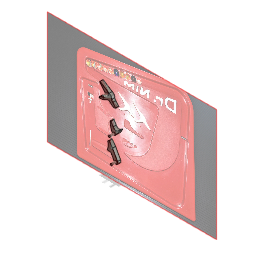
Controls (Autodesk Fusion 360 design; units mm, degrees)
Autodesk Fusion 360 part; units mm, degrees
sketch "Sketch1" plane through (0, 0, 0) normal (0, 0, 1) x (1, 0, 0)
  line L0 (-51.0325, 45.1577) -> (-34.9506, 34.906)
  line L1 (-51.6438, 44.279) -> (-42.8604, 33.3957)
  spline S0 degree 5 poles (-52.4084, 20.9295) (-52.2174, 21.0253) (-51.8369, 21.2159) (-51.271, 21.499) (-50.5262, 21.8709) (-49.6123, 22.3257) (-48.7173, 22.7695) (-47.8428, 23.2013) (-46.9901, 23.6204) (-46.1587, 24.0272) (-45.3471, 24.4223) (-44.7125, 24.7299) (-44.2442, 24.9561) (-43.9354, 25.1049) (-43.7819, 25.1788) knots 0 0 0 0 0 0 0.1 0.2 0.3 0.4 0.5 0.6 0.7 0.8 0.9 1 1 1 1 1 1
  line L2 (-43.6283, 20.7248) -> (-38.8415, 23.1566)
  line L3 (-38.8415, 23.1566) -> (-43.6283, 20.7248)
  line L4 (-28.4743, 24.2061) -> (-23.3292, 18.2162)
  spline S1 degree 5 poles (-42.8604, 33.3957) (-42.7748, 33.2875) (-42.6091, 33.0705) (-42.377, 32.7437) (-42.1008, 32.3051) (-41.8149, 31.7517) (-41.5939, 31.1927) (-41.4431, 30.6277) (-41.3661, 30.0564) (-41.3603, 29.4789) (-41.4207, 28.8958) (-41.5177, 28.4251) (-41.616, 28.0699) (-41.6928, 27.8321) (-41.7341, 27.713) knots 0 0 0 0 0 0 0.1 0.2 0.3 0.4 0.5 0.6 0.7 0.8 0.9 1 1 1 1 1 1
  spline S2 degree 5 poles (-41.7341, 27.713) (-41.759, 27.6465) (-41.8102, 27.515) (-41.8911, 27.3218) (-42.0077, 27.0726) (-42.1685, 26.776) (-42.3458, 26.4956) (-42.5411, 26.2329) (-42.7551, 25.9885) (-42.9871, 25.7619) (-43.2359, 25.5516) (-43.4471, 25.3955) (-43.612, 25.2847) (-43.7248, 25.2136) (-43.7819, 25.1788) knots 0 0 0 0 0 0 0.1 0.2 0.3 0.4 0.5 0.6 0.7 0.8 0.9 1 1 1 1 1 1
  spline S3 degree 5 poles (-43.6283, 20.7248) (-43.7891, 20.6427) (-44.1116, 20.4839) (-44.5982, 20.2616) (-45.2528, 19.9976) (-46.0811, 19.725) (-46.9205, 19.5152) (-47.7719, 19.3729) (-48.6357, 19.301) (-49.5115, 19.2964) (-50.3982, 19.354) (-51.1157, 19.4457) (-51.658, 19.5385) (-52.0214, 19.6108) (-52.2036, 19.6497) knots 0 0 0 0 0 0 0.1 0.2 0.3 0.4 0.5 0.6 0.7 0.8 0.9 1 1 1 1 1 1
  spline S4 degree 5 poles (-52.4084, 20.9295) (-52.4626, 20.896) (-52.5658, 20.8297) (-52.7055, 20.7322) (-52.8605, 20.6065) (-52.9991, 20.4569) (-53.0773, 20.3155) (-53.0905, 20.1829) (-53.0359, 20.0596) (-52.9164, 19.9451) (-52.7369, 19.8387) (-52.5492, 19.7596) (-52.3853, 19.7034) (-52.2658, 19.6673) (-52.2036, 19.6497) knots 0 0 0 0 0 0 0.1 0.2 0.3 0.4 0.5 0.6 0.7 0.8 0.9 1 1 1 1 1 1
  spline S5 degree 5 poles (-38.8415, 23.1566) (-38.7144, 23.2222) (-38.461, 23.3447) (-38.083, 23.5021) (-37.5831, 23.6584) (-36.9658, 23.7583) (-36.3565, 23.7549) (-35.756, 23.6407) (-35.1644, 23.4129) (-34.5812, 23.0779) (-34.0058, 22.6444) (-33.551, 22.2256) (-33.213, 21.8736) (-32.9889, 21.6224) (-32.8772, 21.4927) knots 0 0 0 0 0 0 0.1 0.2 0.3 0.4 0.5 0.6 0.7 0.8 0.9 1 1 1 1 1 1
  spline S6 degree 5 poles (-32.8772, 21.4927) (-32.7115, 21.3178) (-32.3789, 20.9756) (-31.8763, 20.4844) (-31.1986, 19.8749) (-30.3379, 19.1937) (-29.4624, 18.6011) (-28.5707, 18.105) (-27.6619, 17.7112) (-26.7363, 17.4175) (-25.795, 17.2172) (-25.0304, 17.126) (-24.4509, 17.094) (-24.0619, 17.0886) (-23.8667, 17.0899) knots 0 0 0 0 0 0 0.1 0.2 0.3 0.4 0.5 0.6 0.7 0.8 0.9 1 1 1 1 1 1
  spline S7 degree 5 poles (-23.3292, 18.2162) (-23.2856, 18.1711) (-23.2033, 18.083) (-23.094, 17.9567) (-22.9773, 17.8003) (-22.8831, 17.6263) (-22.8451, 17.4756) (-22.8678, 17.3501) (-22.9535, 17.2507) (-23.0996, 17.1764) (-23.3014, 17.1252) (-23.5037, 17.1012) (-23.677, 17.0921) (-23.8019, 17.09) (-23.8667, 17.0899) knots 0 0 0 0 0 0 0.1 0.2 0.3 0.4 0.5 0.6 0.7 0.8 0.9 1 1 1 1 1 1
  spline S8 degree 5 poles (-51.6438, 44.279) (-51.6575, 44.3127) (-51.6828, 44.3788) (-51.7139, 44.4736) (-51.7415, 44.5913) (-51.7512, 44.7232) (-51.7341, 44.8384) (-51.6879, 44.9355) (-51.6115, 45.0139) (-51.5061, 45.0744) (-51.3741, 45.1182) (-51.2489, 45.1411) (-51.1446, 45.1519) (-51.0706, 45.1562) (-51.0325, 45.1577) knots 0 0 0 0 0 0 0.1 0.2 0.3 0.4 0.5 0.6 0.7 0.8 0.9 1 1 1 1 1 1
  spline S9 degree 5 poles (-34.9506, 34.906) (-34.7674, 34.8015) (-34.4087, 34.5894) (-33.894, 34.262) (-33.2553, 33.8065) (-32.5413, 33.2037) (-31.92, 32.5641) (-31.3994, 31.8845) (-30.9854, 31.1626) (-30.6754, 30.3995) (-30.4623, 29.5978) (-30.3633, 28.9281) (-30.3267, 28.4109) (-30.3189, 28.0595) (-30.319, 27.8821) knots 0 0 0 0 0 0 0.1 0.2 0.3 0.4 0.5 0.6 0.7 0.8 0.9 1 1 1 1 1 1
  spline S10 degree 5 poles (-30.319, 27.8821) (-30.3191, 27.8105) (-30.3158, 27.6669) (-30.301, 27.4512) (-30.2612, 27.1624) (-30.1755, 26.7998) (-30.0512, 26.4352) (-29.8854, 26.0685) (-29.6775, 25.6997) (-29.43, 25.329) (-29.1463, 24.9564) (-28.8929, 24.657) (-28.6889, 24.4318) (-28.5469, 24.2814) (-28.4743, 24.2061) knots 0 0 0 0 0 0 0.1 0.2 0.3 0.4 0.5 0.6 0.7 0.8 0.9 1 1 1 1 1 1
  point P0 (-47.6728, 23.2846)
  point P1 (-41.4525, 30.58)
  point P2 (-42.5532, 26.2283)
  point P3 (-47.7496, 19.3937)
  point P4 (-53.0739, 20.1872)
  point P5 (-35.8721, 23.6429)
  point P6 (-28.372, 18.037)
  point P7 (-22.8818, 17.3604)
  point P8 (-51.682, 44.9285)
  point P9 (-31.3427, 31.7457)
  point P10 (-29.9228, 26.165)
  constraint parallel L2 L3
extrude "Extrude1" add sketch "Sketch1" along normal blind 5.5 makes body 1
sketch "Sketch2" plane through (0, 0, 5.5) normal (0, 0, 1) x (1, 0, 0)
  line L0 (-51.6438, 44.279) -> (-42.8604, 33.3957)
  spline S0 degree 5 poles (-42.8604, 33.3957) (-42.7748, 33.2875) (-42.6091, 33.0705) (-42.377, 32.7437) (-42.1008, 32.3051) (-41.8149, 31.7517) (-41.5939, 31.1927) (-41.4431, 30.6277) (-41.3661, 30.0564) (-41.3603, 29.4789) (-41.4207, 28.8958) (-41.5177, 28.4251) (-41.616, 28.0699) (-41.6928, 27.8321) (-41.7341, 27.713) knots 0 0 0 0 0 0 0.1 0.2 0.3 0.4 0.5 0.6 0.7 0.8 0.9 1 1 1 1 1 1
  spline S1 degree 5 poles (-41.7341, 27.713) (-41.759, 27.6465) (-41.8102, 27.515) (-41.8911, 27.3218) (-42.0077, 27.0726) (-42.1685, 26.776) (-42.3458, 26.4956) (-42.5411, 26.2329) (-42.7551, 25.9885) (-42.9871, 25.7619) (-43.2359, 25.5516) (-43.4471, 25.3955) (-43.612, 25.2847) (-43.7248, 25.2136) (-43.7819, 25.1788) knots 0 0 0 0 0 0 0.1 0.2 0.3 0.4 0.5 0.6 0.7 0.8 0.9 1 1 1 1 1 1
  spline S2 degree 5 poles (-43.7819, 25.1788) (-43.9354, 25.1049) (-44.2442, 24.9561) (-44.7125, 24.7299) (-45.3471, 24.4223) (-46.1587, 24.0272) (-46.9901, 23.6204) (-47.8428, 23.2013) (-48.7173, 22.7695) (-49.6123, 22.3257) (-50.5262, 21.8709) (-51.271, 21.499) (-51.8369, 21.2159) (-52.2174, 21.0253) (-52.4084, 20.9295) knots -1 -1 -1 -1 -1 -1 -0.9 -0.8 -0.7 -0.6 -0.5 -0.4 -0.3 -0.2 -0.1 0 0 0 0 0 0
  spline S3 degree 5 poles (-52.4084, 20.9295) (-52.4626, 20.896) (-52.5658, 20.8297) (-52.7055, 20.7322) (-52.8605, 20.6065) (-52.9991, 20.4569) (-53.0773, 20.3155) (-53.0905, 20.1829) (-53.0359, 20.0596) (-52.9164, 19.9451) (-52.7369, 19.8387) (-52.5492, 19.7596) (-52.3853, 19.7034) (-52.2658, 19.6673) (-52.2036, 19.6497) knots 0 0 0 0 0 0 0.1 0.2 0.3 0.4 0.5 0.6 0.7 0.8 0.9 1 1 1 1 1 1
  spline S4 degree 5 poles (-52.2036, 19.6497) (-52.0214, 19.6108) (-51.658, 19.5385) (-51.1157, 19.4457) (-50.3982, 19.354) (-49.5115, 19.2964) (-48.6357, 19.301) (-47.7719, 19.3729) (-46.9205, 19.5152) (-46.0811, 19.725) (-45.2528, 19.9976) (-44.5982, 20.2616) (-44.1116, 20.4839) (-43.7891, 20.6427) (-43.6283, 20.7248) knots -1 -1 -1 -1 -1 -1 -0.9 -0.8 -0.7 -0.6 -0.5 -0.4 -0.3 -0.2 -0.1 0 0 0 0 0 0
  line L1 (-43.6283, 20.7248) -> (-38.8415, 23.1566)
  spline S5 degree 5 poles (-38.8415, 23.1566) (-38.7144, 23.2222) (-38.461, 23.3447) (-38.083, 23.5021) (-37.5831, 23.6584) (-36.9658, 23.7583) (-36.3565, 23.7549) (-35.756, 23.6407) (-35.1644, 23.4129) (-34.5812, 23.0779) (-34.0058, 22.6444) (-33.551, 22.2256) (-33.213, 21.8736) (-32.9889, 21.6224) (-32.8772, 21.4927) knots 0 0 0 0 0 0 0.1 0.2 0.3 0.4 0.5 0.6 0.7 0.8 0.9 1 1 1 1 1 1
  spline S6 degree 5 poles (-32.8772, 21.4927) (-32.7115, 21.3178) (-32.3789, 20.9756) (-31.8763, 20.4844) (-31.1986, 19.8749) (-30.3379, 19.1937) (-29.4624, 18.6011) (-28.5707, 18.105) (-27.6619, 17.7112) (-26.7363, 17.4175) (-25.795, 17.2172) (-25.0304, 17.126) (-24.4509, 17.094) (-24.0619, 17.0886) (-23.8667, 17.0899) knots 0 0 0 0 0 0 0.1 0.2 0.3 0.4 0.5 0.6 0.7 0.8 0.9 1 1 1 1 1 1
  spline S7 degree 5 poles (-23.8667, 17.0899) (-23.8019, 17.09) (-23.677, 17.0921) (-23.5037, 17.1012) (-23.3014, 17.1252) (-23.0996, 17.1764) (-22.9535, 17.2507) (-22.8678, 17.3501) (-22.8451, 17.4756) (-22.8831, 17.6263) (-22.9773, 17.8003) (-23.094, 17.9567) (-23.2033, 18.083) (-23.2856, 18.1711) (-23.3292, 18.2162) knots -1 -1 -1 -1 -1 -1 -0.9 -0.8 -0.7 -0.6 -0.5 -0.4 -0.3 -0.2 -0.1 0 0 0 0 0 0
  line L2 (-23.3292, 18.2162) -> (-28.4743, 24.2061)
  spline S8 degree 5 poles (-28.4743, 24.2061) (-28.5469, 24.2814) (-28.6889, 24.4318) (-28.8929, 24.657) (-29.1463, 24.9564) (-29.43, 25.329) (-29.6775, 25.6997) (-29.8854, 26.0685) (-30.0512, 26.4352) (-30.1755, 26.7998) (-30.2612, 27.1624) (-30.301, 27.4512) (-30.3158, 27.6669) (-30.3191, 27.8105) (-30.319, 27.8821) knots -1 -1 -1 -1 -1 -1 -0.9 -0.8 -0.7 -0.6 -0.5 -0.4 -0.3 -0.2 -0.1 0 0 0 0 0 0
  spline S9 degree 5 poles (-30.319, 27.8821) (-30.3189, 28.0595) (-30.3267, 28.4109) (-30.3633, 28.9281) (-30.4623, 29.5978) (-30.6754, 30.3995) (-30.9854, 31.1626) (-31.3994, 31.8845) (-31.92, 32.5641) (-32.5413, 33.2037) (-33.2553, 33.8065) (-33.894, 34.262) (-34.4087, 34.5894) (-34.7674, 34.8015) (-34.9506, 34.906) knots -1 -1 -1 -1 -1 -1 -0.9 -0.8 -0.7 -0.6 -0.5 -0.4 -0.3 -0.2 -0.1 0 0 0 0 0 0
  line L3 (-34.9506, 34.906) -> (-51.0325, 45.1577)
  spline S10 degree 5 poles (-51.0325, 45.1577) (-51.0706, 45.1562) (-51.1446, 45.1519) (-51.2489, 45.1411) (-51.3741, 45.1182) (-51.5061, 45.0744) (-51.6115, 45.0139) (-51.6879, 44.9355) (-51.7341, 44.8384) (-51.7512, 44.7232) (-51.7415, 44.5913) (-51.7139, 44.4736) (-51.6828, 44.3788) (-51.6575, 44.3127) (-51.6438, 44.279) knots -1 -1 -1 -1 -1 -1 -0.9 -0.8 -0.7 -0.6 -0.5 -0.4 -0.3 -0.2 -0.1 0 0 0 0 0 0
  circle A0 centre (-37.8334, 32.2567) radius 1.9
  dimension "d3" = 3.8
  measures "d3" diameter of A0
extrude "Extrude2" add sketch "Sketch2" along normal blind 4.5 contours A0 bodies 1
sketch "Sketch3" plane through (0, 0, 0) normal (0, 0, 1) x (1, 0, 0)
  spline S0 degree 5 poles (-32.9136, -6.4027) (-32.9211, -6.7481) (-32.929, -7.4377) (-32.919, -8.4686) (-32.8613, -9.8362) (-32.7103, -11.533) (-32.4735, -13.2163) (-32.144, -14.8848) (-31.7181, -16.538) (-31.2001, -18.1766) (-30.5969, -19.8016) (-30.0518, -21.0916) (-29.6101, -22.054) (-29.3013, -22.6933) (-29.1433, -23.0123) knots 0 0 0 0 0 0 0.1 0.2 0.3 0.4 0.5 0.6 0.7 0.8 0.9 1 1 1 1 1 1
  spline S1 degree 5 poles (-23.9464, -23.8954) (-23.7767, -23.7611) (-23.4398, -23.487) (-22.9418, -23.0601) (-22.2929, -22.4586) (-21.5087, -21.6493) (-20.7535, -20.7781) (-20.0294, -19.8404) (-19.337, -18.835) (-18.6744, -17.7659) (-18.0391, -16.6384) (-17.5508, -15.6938) (-17.1951, -14.963) (-16.9625, -14.4659) (-16.8474, -14.215) knots 0 0 0 0 0 0 0.1 0.2 0.3 0.4 0.5 0.6 0.7 0.8 0.9 1 1 1 1 1 1
  spline S2 degree 5 poles (-29.1433, -23.0123) (-29.0398, -23.1384) (-28.8329, -23.3813) (-28.5224, -23.7176) (-28.1081, -24.1092) (-27.5898, -24.4975) (-27.0709, -24.775) (-26.5516, -24.9318) (-26.0316, -24.9612) (-25.5111, -24.8662) (-24.99, -24.6553) (-24.5728, -24.4012) (-24.2597, -24.1656) (-24.0508, -23.9888) (-23.9464, -23.8954) knots 0 0 0 0 0 0 0.1 0.2 0.3 0.4 0.5 0.6 0.7 0.8 0.9 1 1 1 1 1 1
  line L0 (-31.6568, -6.063) -> (-27.7846, -12.8903)
  spline S3 degree 5 poles (-27.7846, -12.8903) (-27.6213, -13.1416) (-27.2915, -13.6236) (-26.7879, -14.285) (-26.098, -15.0415) (-25.2028, -15.7641) (-24.272, -16.2445) (-23.3028, -16.4635) (-22.2938, -16.4123) (-21.247, -16.1031) (-20.1652, -15.5563) (-19.2742, -14.9446) (-18.5924, -14.3941) (-18.132, -13.987) (-17.9004, -13.7734) knots 0 0 0 0 0 0 0.1 0.2 0.3 0.4 0.5 0.6 0.7 0.8 0.9 1 1 1 1 1 1
  spline S4 degree 5 poles (-17.9004, -13.7734) (-17.8375, -13.7089) (-17.7155, -13.5863) (-17.5433, -13.4214) (-17.3358, -13.2404) (-17.1159, -13.0833) (-16.9389, -13.0016) (-16.8084, -13.0016) (-16.7268, -13.0874) (-16.6924, -13.2559) (-16.7016, -13.5011) (-16.7412, -13.7538) (-16.7878, -13.973) (-16.8263, -14.1322) (-16.8474, -14.215) knots 0 0 0 0 0 0 0.1 0.2 0.3 0.4 0.5 0.6 0.7 0.8 0.9 1 1 1 1 1 1
  spline S5 degree 5 poles (-32.9136, -6.4027) (-32.9127, -6.3184) (-32.9088, -6.1566) (-32.8967, -5.9343) (-32.8676, -5.6793) (-32.8081, -5.4341) (-32.7234, -5.269) (-32.6117, -5.1906) (-32.4718, -5.2021) (-32.3049, -5.2998) (-32.113, -5.4771) (-31.9412, -5.6774) (-31.8027, -5.8585) (-31.7061, -5.9926) (-31.6568, -6.063) knots 0 0 0 0 0 0 0.1 0.2 0.3 0.4 0.5 0.6 0.7 0.8 0.9 1 1 1 1 1 1
  point P0 (-32.1323, -14.8264)
  point P1 (-20.2101, -20.0572)
  point P2 (-26.4599, -24.9144)
  point P3 (-23.369, -16.3888)
  point P4 (-16.8134, -13.0262)
  point P5 (-32.6079, -5.2139)
extrude "Extrude3" add sketch "Sketch3" along normal blind 5.5 separate body makes body 2
sketch "Sketch4" plane through (0, 0, 5.5) normal (0, 0, 1) x (1, 0, 0)
  spline S0 degree 5 poles (-29.1433, -23.0123) (-29.0398, -23.1384) (-28.8329, -23.3813) (-28.5224, -23.7176) (-28.1081, -24.1092) (-27.5898, -24.4975) (-27.0709, -24.775) (-26.5516, -24.9318) (-26.0316, -24.9612) (-25.5111, -24.8662) (-24.99, -24.6553) (-24.5728, -24.4012) (-24.2597, -24.1656) (-24.0508, -23.9888) (-23.9464, -23.8954) knots 0 0 0 0 0 0 0.1 0.2 0.3 0.4 0.5 0.6 0.7 0.8 0.9 1 1 1 1 1 1
  spline S1 degree 5 poles (-23.9464, -23.8954) (-23.7767, -23.7611) (-23.4398, -23.487) (-22.9418, -23.0601) (-22.2929, -22.4586) (-21.5087, -21.6493) (-20.7535, -20.7781) (-20.0294, -19.8404) (-19.337, -18.835) (-18.6744, -17.7659) (-18.0391, -16.6384) (-17.5508, -15.6938) (-17.1951, -14.963) (-16.9625, -14.4659) (-16.8474, -14.215) knots 0 0 0 0 0 0 0.1 0.2 0.3 0.4 0.5 0.6 0.7 0.8 0.9 1 1 1 1 1 1
  spline S2 degree 5 poles (-16.8474, -14.215) (-16.8263, -14.1322) (-16.7878, -13.973) (-16.7412, -13.7538) (-16.7016, -13.5011) (-16.6924, -13.2559) (-16.7268, -13.0874) (-16.8084, -13.0016) (-16.9389, -13.0016) (-17.1159, -13.0833) (-17.3358, -13.2404) (-17.5433, -13.4214) (-17.7155, -13.5863) (-17.8375, -13.7089) (-17.9004, -13.7734) knots -1 -1 -1 -1 -1 -1 -0.9 -0.8 -0.7 -0.6 -0.5 -0.4 -0.3 -0.2 -0.1 0 0 0 0 0 0
  spline S3 degree 5 poles (-17.9004, -13.7734) (-18.132, -13.987) (-18.5924, -14.3941) (-19.2742, -14.9446) (-20.1652, -15.5563) (-21.247, -16.1031) (-22.2938, -16.4123) (-23.3028, -16.4635) (-24.272, -16.2445) (-25.2028, -15.7641) (-26.098, -15.0415) (-26.7879, -14.285) (-27.2915, -13.6236) (-27.6213, -13.1416) (-27.7846, -12.8903) knots -1 -1 -1 -1 -1 -1 -0.9 -0.8 -0.7 -0.6 -0.5 -0.4 -0.3 -0.2 -0.1 0 0 0 0 0 0
  line L0 (-27.7846, -12.8903) -> (-31.6568, -6.063)
  spline S4 degree 5 poles (-31.6568, -6.063) (-31.7061, -5.9926) (-31.8027, -5.8585) (-31.9412, -5.6774) (-32.113, -5.4771) (-32.3049, -5.2998) (-32.4718, -5.2021) (-32.6117, -5.1906) (-32.7234, -5.269) (-32.8081, -5.4341) (-32.8676, -5.6793) (-32.8967, -5.9343) (-32.9088, -6.1566) (-32.9127, -6.3184) (-32.9136, -6.4027) knots -1 -1 -1 -1 -1 -1 -0.9 -0.8 -0.7 -0.6 -0.5 -0.4 -0.3 -0.2 -0.1 0 0 0 0 0 0
  spline S5 degree 5 poles (-32.9136, -6.4027) (-32.9211, -6.7481) (-32.929, -7.4377) (-32.919, -8.4686) (-32.8613, -9.8362) (-32.7103, -11.533) (-32.4735, -13.2163) (-32.144, -14.8848) (-31.7181, -16.538) (-31.2001, -18.1766) (-30.5969, -19.8016) (-30.0518, -21.0916) (-29.6101, -22.054) (-29.3013, -22.6933) (-29.1433, -23.0123) knots 0 0 0 0 0 0 0.1 0.2 0.3 0.4 0.5 0.6 0.7 0.8 0.9 1 1 1 1 1 1
  circle A0 centre (-26.0929, -22.3583) radius 1.9
  dimension "d8" = 3.8
  measures "d8" diameter of A0
extrude "Extrude4" add sketch "Sketch4" along normal blind 4.5 contours A0 bodies 2
sketch "Sketch5" plane through (0, 0, 0) normal (0, 0, 1) x (1, 0, 0)
  line L0 (-28.8892, -46.1495) -> (-20.1605, -62.1427)
  line L1 (-31.2219, -55.2328) -> (-25.6392, -65.5712)
  spline S0 degree 5 poles (-25.6392, -65.5712) (-25.5584, -65.6892) (-25.3954, -65.9179) (-25.1471, -66.2389) (-24.8079, -66.6222) (-24.3697, -67.0214) (-23.9159, -67.3334) (-23.4451, -67.5505) (-22.9564, -67.6676) (-22.4503, -67.6874) (-21.9281, -67.6166) (-21.4983, -67.4933) (-21.1697, -67.3656) (-20.9479, -67.2651) (-20.8363, -67.211) knots 0 0 0 0 0 0 0.1 0.2 0.3 0.4 0.5 0.6 0.7 0.8 0.9 1 1 1 1 1 1
  spline S1 degree 5 poles (-20.1605, -62.1427) (-20.1013, -62.2647) (-19.9893, -62.5069) (-19.84, -62.8648) (-19.6792, -63.3312) (-19.5465, -63.8948) (-19.4882, -64.4373) (-19.5109, -64.9569) (-19.6187, -65.4523) (-19.8094, -65.9242) (-20.0769, -66.3743) (-20.3476, -66.7184) (-20.5805, -66.9679) (-20.7488, -67.1306) (-20.8363, -67.211) knots 0 0 0 0 0 0 0.1 0.2 0.3 0.4 0.5 0.6 0.7 0.8 0.9 1 1 1 1 1 1
  spline S2 degree 5 poles (-28.8892, -46.1495) (-29.0126, -45.9468) (-29.2593, -45.5447) (-29.6296, -44.9516) (-30.1236, -44.1813) (-30.7416, -43.2549) (-31.3601, -42.3684) (-31.9792, -41.5258) (-32.599, -40.7297) (-33.2193, -39.9795) (-33.8402, -39.2724) (-34.3374, -38.7384) (-34.7105, -38.3548) (-34.9593, -38.1063) (-35.0838, -37.9839) knots 0 0 0 0 0 0 0.1 0.2 0.3 0.4 0.5 0.6 0.7 0.8 0.9 1 1 1 1 1 1
  spline S3 degree 5 poles (-37.3216, -39.4151) (-37.2534, -39.6592) (-37.124, -40.1484) (-36.9506, -40.8848) (-36.7615, -41.872) (-36.6002, -43.1154) (-36.5203, -44.3691) (-36.5283, -45.6339) (-36.6269, -46.9101) (-36.8118, -48.1973) (-37.0762, -49.4945) (-37.3461, -50.5396) (-37.5791, -51.3273) (-37.7479, -51.8541) (-37.8356, -52.118) knots 0 0 0 0 0 0 0.1 0.2 0.3 0.4 0.5 0.6 0.7 0.8 0.9 1 1 1 1 1 1
  spline S4 degree 5 poles (-37.3216, -39.4151) (-37.3222, -39.3189) (-37.3194, -39.1324) (-37.3034, -38.8704) (-37.2579, -38.5571) (-37.1578, -38.2297) (-37.0109, -37.9722) (-36.8132, -37.7901) (-36.5629, -37.6866) (-36.262, -37.6583) (-35.9144, -37.6996) (-35.6021, -37.7836) (-35.3498, -37.8735) (-35.1738, -37.9452) (-35.0838, -37.9839) knots 0 0 0 0 0 0 0.1 0.2 0.3 0.4 0.5 0.6 0.7 0.8 0.9 1 1 1 1 1 1
  line L2 (-36.6879, -53.8517) -> (-33.8553, -53.5831)
  spline S5 degree 5 poles (-37.8356, -52.118) (-37.8715, -52.202) (-37.9381, -52.3659) (-38.0228, -52.5988) (-38.1046, -52.8834) (-38.1516, -53.1926) (-38.1382, -53.4511) (-38.0592, -53.6545) (-37.9114, -53.8001) (-37.697, -53.8898) (-37.4207, -53.9276) (-37.1541, -53.9195) (-36.9302, -53.8933) (-36.7704, -53.8671) (-36.6879, -53.8517) knots 0 0 0 0 0 0 0.1 0.2 0.3 0.4 0.5 0.6 0.7 0.8 0.9 1 1 1 1 1 1
  spline S6 degree 5 poles (-33.8553, -53.5831) (-33.7801, -53.5674) (-33.6316, -53.5402) (-33.4148, -53.5124) (-33.1379, -53.5014) (-32.8133, -53.5342) (-32.5121, -53.6177) (-32.2363, -53.7557) (-31.9865, -53.9499) (-31.7616, -54.1978) (-31.5596, -54.4951) (-31.4148, -54.7691) (-31.315, -54.9937) (-31.2523, -55.1517) (-31.2219, -55.2328) knots 0 0 0 0 0 0 0.1 0.2 0.3 0.4 0.5 0.6 0.7 0.8 0.9 1 1 1 1 1 1
  point P0 (-23.3704, -67.5489)
  point P1 (-19.541, -65.0148)
  point P2 (-32.1554, -41.3065)
  point P3 (-36.5462, -45.5147)
  point P4 (-36.8046, -37.8126)
  point P5 (-38.031, -53.6564)
  point P6 (-32.2681, -53.754)
extrude "Extrude5" add sketch "Sketch5" along normal blind 5.5 separate body makes body 3
sketch "Sketch6" plane through (0, 0, 5.5) normal (0, 0, 1) x (1, 0, 0)
  spline S0 degree 5 poles (-37.3216, -39.4151) (-37.2534, -39.6592) (-37.124, -40.1484) (-36.9506, -40.8848) (-36.7615, -41.872) (-36.6002, -43.1154) (-36.5203, -44.3691) (-36.5283, -45.6339) (-36.6269, -46.9101) (-36.8118, -48.1973) (-37.0762, -49.4945) (-37.3461, -50.5396) (-37.5791, -51.3273) (-37.7479, -51.8541) (-37.8356, -52.118) knots 0 0 0 0 0 0 0.1 0.2 0.3 0.4 0.5 0.6 0.7 0.8 0.9 1 1 1 1 1 1
  spline S1 degree 5 poles (-37.8356, -52.118) (-37.8715, -52.202) (-37.9381, -52.3659) (-38.0228, -52.5988) (-38.1046, -52.8834) (-38.1516, -53.1926) (-38.1382, -53.4511) (-38.0592, -53.6545) (-37.9114, -53.8001) (-37.697, -53.8898) (-37.4207, -53.9276) (-37.1541, -53.9195) (-36.9302, -53.8933) (-36.7704, -53.8671) (-36.6879, -53.8517) knots 0 0 0 0 0 0 0.1 0.2 0.3 0.4 0.5 0.6 0.7 0.8 0.9 1 1 1 1 1 1
  line L0 (-36.6879, -53.8517) -> (-33.8553, -53.5831)
  spline S2 degree 5 poles (-33.8553, -53.5831) (-33.7801, -53.5674) (-33.6316, -53.5402) (-33.4148, -53.5124) (-33.1379, -53.5014) (-32.8133, -53.5342) (-32.5121, -53.6177) (-32.2363, -53.7557) (-31.9865, -53.9499) (-31.7616, -54.1978) (-31.5596, -54.4951) (-31.4148, -54.7691) (-31.315, -54.9937) (-31.2523, -55.1517) (-31.2219, -55.2328) knots 0 0 0 0 0 0 0.1 0.2 0.3 0.4 0.5 0.6 0.7 0.8 0.9 1 1 1 1 1 1
  line L1 (-31.2219, -55.2328) -> (-25.6392, -65.5712)
  spline S3 degree 5 poles (-25.6392, -65.5712) (-25.5584, -65.6892) (-25.3954, -65.9179) (-25.1471, -66.2389) (-24.8079, -66.6222) (-24.3697, -67.0214) (-23.9159, -67.3334) (-23.4451, -67.5505) (-22.9564, -67.6676) (-22.4503, -67.6874) (-21.9281, -67.6166) (-21.4983, -67.4933) (-21.1697, -67.3656) (-20.9479, -67.2651) (-20.8363, -67.211) knots 0 0 0 0 0 0 0.1 0.2 0.3 0.4 0.5 0.6 0.7 0.8 0.9 1 1 1 1 1 1
  spline S4 degree 5 poles (-20.8363, -67.211) (-20.7488, -67.1306) (-20.5805, -66.9679) (-20.3476, -66.7184) (-20.0769, -66.3743) (-19.8094, -65.9242) (-19.6187, -65.4523) (-19.5109, -64.9569) (-19.4882, -64.4373) (-19.5465, -63.8948) (-19.6792, -63.3312) (-19.84, -62.8648) (-19.9893, -62.5069) (-20.1013, -62.2647) (-20.1605, -62.1427) knots -1 -1 -1 -1 -1 -1 -0.9 -0.8 -0.7 -0.6 -0.5 -0.4 -0.3 -0.2 -0.1 0 0 0 0 0 0
  line L2 (-20.1605, -62.1427) -> (-28.8892, -46.1495)
  spline S5 degree 5 poles (-28.8892, -46.1495) (-29.0126, -45.9468) (-29.2593, -45.5447) (-29.6296, -44.9516) (-30.1236, -44.1813) (-30.7416, -43.2549) (-31.3601, -42.3684) (-31.9792, -41.5258) (-32.599, -40.7297) (-33.2193, -39.9795) (-33.8402, -39.2724) (-34.3374, -38.7384) (-34.7105, -38.3548) (-34.9593, -38.1063) (-35.0838, -37.9839) knots 0 0 0 0 0 0 0.1 0.2 0.3 0.4 0.5 0.6 0.7 0.8 0.9 1 1 1 1 1 1
  spline S6 degree 5 poles (-35.0838, -37.9839) (-35.1738, -37.9452) (-35.3498, -37.8735) (-35.6021, -37.7836) (-35.9144, -37.6996) (-36.262, -37.6583) (-36.5629, -37.6866) (-36.8132, -37.7901) (-37.0109, -37.9722) (-37.1578, -38.2297) (-37.2579, -38.5571) (-37.3034, -38.8704) (-37.3194, -39.1324) (-37.3222, -39.3189) (-37.3216, -39.4151) knots -1 -1 -1 -1 -1 -1 -0.9 -0.8 -0.7 -0.6 -0.5 -0.4 -0.3 -0.2 -0.1 0 0 0 0 0 0
  circle A0 centre (-22.7852, -63.8704) radius 1.9
  dimension "d13" = 3.8
  measures "d13" diameter of A0
extrude "Extrude6" add sketch "Sketch6" along normal blind 4.5 contours A0 bodies 3
extrude "Extrude7" add 1 faces at (-38.404, 32.5315, 10) along direction (0, 0, 1) blind 3.5 on bodies 1 bodies 1
extrude "Extrude8" add 1 faces at (-26.5978, -22.9209, 10) along direction (0, 0, 1) blind 1.5 on bodies 2 bodies 2
extrude "Extrude9" add 1 faces at (-23.9039, -64.1862, 10) along direction (0, 0, 1) blind 1.5 on bodies 3 bodies 3
extrude "Extrude10" add 1 faces at (-23.9039, -64.1862, 11.5) along direction (0, 0, 1) blind 2.5 on bodies 3 bodies 3
extrude "Extrude11" add 1 faces at (-26.5978, -22.9209, 11.5) along direction (0, 0, 1) blind 2.5 on bodies 2 bodies 2
